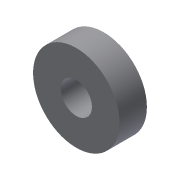
# Autodesk Inventor part: BallBearing
Saved by Autodesk Inventor 2015 (Build 190159000, 159)
## iProperties
Created: 2015-01-18
Part Number: BallBearing
Material: Generic
Document SubType Name: Modeling
Designer: Tanner
Density: 1 g/cm^3
Appearance: Default
Author: Tanner
Autodesk Inventor part; units mm, degrees
ref_plane "YZ Plane" through (0, 0, 0) normal (1, 0, 0) x (0, 1, 0)
ref_plane "XZ Plane" through (0, 0, 0) normal (0, 1, 0) x (-1, 0, 0)
ref_plane "XY Plane" through (0, 0, 0) normal (0, 0, 1) x (1, 0, 0)
sketch "Sketch1" plane through (0, 0, 0) normal (0, 0, 1) x (1, 0, 0)
  circle A0 centre (0, 0) radius 10.9474
  circle A1 centre (0, 0) radius 3.9624
  dimension "d0" = 21.8948
  dimension "d1" = 7.9248
  constraints: 2 centre point, 2 coincident
  measures "d0" diameter of A0
  measures "d1" diameter of A1
extrude "Extrusion1" add sketch "Sketch1" along normal blind 6.9342
body "Solid1"
